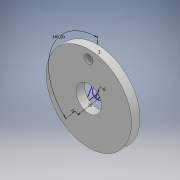
# Autodesk Inventor part: test wysiegu sprezyny
Saved by Autodesk Inventor 2017 (Build 210142000, 142)
## iProperties
Created: 2021-05-20
Part Number: test wysiegu sprezyny
Material: Generic
Document SubType Name: Modeling
Designer: majch
Density: 1 g/cm^3
Appearance: Default
Author: majch
Autodesk Inventor part; units mm, degrees
ref_plane "YZ Plane" through (0, 0, 0) normal (1, 0, 0) x (0, 1, 0)
ref_plane "XZ Plane" through (0, 0, 0) normal (0, 1, 0) x (-1, 0, 0)
ref_plane "XY Plane" through (0, 0, 0) normal (0, 0, 1) x (1, 0, 0)
sketch "Sketch1" plane through (0, 0, 0) normal (0, 1, 0) x (-1, 0, 0)
  circle A0 centre (0, 0) radius 25
  dimension "d0" = 50
  constraints: 1 centre point, 1 coincident
  measures "d0" diameter of A0
extrude "Extrusion1" add sketch "Sketch1" along normal blind 5
sketch "Sketch2" plane through (0, 5, 0) normal (0, 1, 0) x (1, 0, 0)
  circle A0 centre (0, 0) radius 7.5
  dimension "d3" = 15
  constraints: 1 centre point, 1 coincident
  measures "d3" diameter of A0
extrude "Extrusion2" cut sketch "Sketch2" against normal through all
sketch "Sketch3" plane through (0, 5, 0) normal (0, 1, 0) x (1, 0, 0)
  circle A0 centre (0, 0) radius 20 construction
  constraints: 1 centre point, 1 coincident
sketch "Sketch4" plane through (0, 5, 0) normal (0, 1, 0) x (1, 0, 0)
  circle A0 centre (0, -20) radius 2.5
  point P0 (0, 0)
  dimension "d8" = 5
  constraints: 1 centre point
  measures "d8" diameter of A0
extrude "Extrusion3" cut sketch "Sketch4" against normal through all
sketch "Sketch5" plane through (0, 5, 0) normal (0, 1, 0) x (1, 0, 0)
  line L0 (0, 0) -> (-12.8558, 15.3209)
  line L1 (0, 0) -> (0, -27.4763)
  arc A0 (-10.0367, 16.3469) -> (-15.6748, 14.2948) centre (-12.8558, 15.3209) ccw
  arc A1 (-2.8191, -21.0261) -> (2.8191, -18.9739) centre (0, -20) ccw
  line L2 (-10.0367, 16.3469) -> (2.8191, -18.9739)
  line L3 (-2.8191, -21.0261) -> (-15.6748, 14.2948)
  circle A2 centre (0, 0) radius 3
  dimension "d11" = 140
  dimension "d14" = 20
  dimension "d15" = 3
  dimension "d17" = 3
  dimension "d18" = 6
  constraints: 8 end point, 4 point on circle, 4 tangent, 3 centre point, 2 coincident, 1 point on line, 1 vertical, 1 other
  measures "d11" angle of L1 L0
  measures "d14" distance of L0.start L0.end
  measures "d15" radius of A1
  measures "d17" radius of A0
  measures "d18" diameter of A2
body "Solid1"
